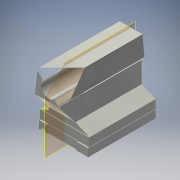
# Autodesk Inventor part: tail stock
Saved by Autodesk Inventor 2016 (Build 200138000, 138)
## iProperties
Created: 2017-02-14
Part Number: tail stock
Material: Steel
Document SubType Name: Modeling
Designer: m207653
Density: 7.85 g/cm^3
Appearance: Smooth - Ivory
Author: m207653
Autodesk Inventor part; units mm, degrees
ref_plane "YZ Plane" through (0, 0, 0) normal (1, 0, 0) x (0, 1, 0)
ref_plane "XZ Plane" through (0, 0, 0) normal (0, 1, 0) x (-1, 0, 0)
ref_plane "XY Plane" through (0, 0, 0) normal (0, 0, 1) x (1, 0, 0)
sketch "Sketch1" plane through (0, 0, 0) normal (0, 1, 0) x (-1, 0, 0)
  line L0 (-14.8781, 49.9341) -> (-14.8781, 23.9341)
  line L1 (-14.8781, 23.9341) -> (-165.8781, 23.9341)
  line L2 (-165.8781, 23.9341) -> (-165.8781, 49.9341)
  line L3 (-165.8781, 49.9341) -> (-14.8781, 49.9341)
  point P0 (0, 0)
  dimension "d19" = 26
  dimension "d20" = 151
  constraints: 8 end point, 3 perpendicular, 1 vertical
  measures "d19" distance of L0.start L0.end
  measures "d20" distance of L0.end L1.end
extrude "Extrusion1" add sketch "Sketch1" along normal blind 203
sketch "Sketch2" plane through (0, 0, 0) normal (0, -1, 0) x (1, 0, 0)
  line L0 (14.8781, 23.9341) -> (14.8781, 49.9341) projected
  line L1 (14.8781, 49.9341) -> (14.8781, 23.9341)
  line L2 (14.8781, 49.9341) -> (42.8781, 49.9341)
  line L3 (14.8781, 49.9341) -> (165.8781, 49.9341) projected
  line L4 (42.8781, 49.9341) -> (42.8781, 23.9341)
  line L5 (165.8781, 23.9341) -> (14.8781, 23.9341) projected
  line L6 (14.8781, 23.9341) -> (42.8781, 23.9341)
  line L7 (27.3781, 49.9341) -> (27.3781, 33.9341) construction
  line L8 (25.4781, 33.9341) -> (38.7147, 33.9341) construction
  line L9 (29.4781, 36.9341) -> (43.9589, 36.9341) construction
  line L10 (27.3781, 33.9341) -> (30.8781, 33.9341)
  line L11 (30.8781, 33.9341) -> (26.8781, 33.9341)
  line L12 (26.8781, 33.9341) -> (16.8781, 23.9341)
  line L13 (26.8781, 33.9341) -> (51.2693, 33.9341) construction
  line L14 (30.8781, 33.9341) -> (40.8781, 23.9341)
  line L15 (30.8781, 33.9341) -> (59.3837, 33.9341) construction
  point P0 (0, 0)
  dimension "d23" = 28
  dimension "d29" = 4
  dimension "d30" = 135
  dimension "d31" = 45
  dimension "d32" = 10
  dimension "d117" = 2
  constraints: 26 end point, 9 point on line, 4 horizontal, 2 collinear, 1 perpendicular
  measures "d23" distance of L0.end L2.end
  measures "d29" distance of L10.end L11.end
  measures "d30" angle of L12 L13
  measures "d31" angle of L14 L15
  measures "d32" vertical distance of L0.start L11.end
  measures "d117" distance of L0.start L12.end
extrude "Extrusion2" cut sketch "Sketch2" against normal through all contours L12 L11 L10 L14 L5
sketch "Sketch3" plane through (0, 0, 0) normal (0, -1, 0) x (1, 0, 0)
  line L0 (14.8781, 23.9341) -> (16.8781, 23.9341) projected
  line L1 (14.8781, 49.9341) -> (14.8781, 23.9341) projected
  line L2 (14.8781, 23.9341) -> (14.8781, 49.9341)
  line L3 (14.8781, 49.9341) -> (42.8781, 49.9341)
  line L4 (165.8781, 49.9341) -> (14.8781, 49.9341) projected
  line L5 (42.8781, 49.9341) -> (42.8781, 23.9341)
  line L6 (40.8781, 23.9341) -> (165.8781, 23.9341) projected
  line L7 (14.8781, 23.9341) -> (16.8781, 23.9341)
  line L8 (16.8781, 23.9341) -> (26.8781, 33.9341) projected
  line L9 (26.8781, 33.9341) -> (16.8781, 23.9341)
  line L10 (16.8781, 23.9341) -> (26.8781, 33.9341)
  line L11 (26.8781, 33.9341) -> (30.8781, 33.9341) projected
  line L12 (30.8781, 33.9341) -> (40.8781, 23.9341) projected
  line L13 (30.8781, 33.9341) -> (40.8781, 23.9341)
  line L14 (40.8781, 23.9341) -> (42.8781, 23.9341)
  point P0 (0, 0)
  dimension "d35" = 28
  constraints: 16 end point, 3 collinear, 2 point on line, 1 horizontal, 1 perpendicular, 1 vertical
  measures "d35" distance of L1.start L3.end
extrude "Extrusion3" add sketch "Sketch3" along normal blind 6
sketch "Sketch4" plane through (14.8781, 203, 49.9341) normal (0, 0, 1) x (1, 0, 0)
  line L0 (0, -209) -> (0, -203)
  line L1 (2, 0) -> (2, -209) projected
  line L2 (151, -203) -> (28, -203) projected
  line L3 (0, -203) -> (28, -203)
  line L4 (28, -209) -> (0, -209) projected
  line L5 (28, -203) -> (28, -209)
  line L6 (28, -209) -> (0, -209)
  line L7 (0, -209) -> (0, -203)
  point P0 (-14.8781, -203)
  constraints: 10 end point, 3 perpendicular, 1 collinear, 1 parallel
extrude "Extrusion4" cut sketch "Sketch4" against normal blind 2
sketch "Sketch5" plane through (0, 0, 0) normal (0, -1, 0) x (1, 0, 0)
  line L0 (165.8781, 23.9341) -> (40.8781, 23.9341) projected
  line L1 (165.8781, 23.9341) -> (165.8781, 47.9341)
  line L2 (165.8781, 49.9341) -> (165.8781, 23.9341) projected
  line L3 (42.8781, 47.9341) -> (14.8781, 47.9341) projected
  line L4 (165.8781, 47.9341) -> (128.8781, 47.9341)
  line L5 (128.8781, 47.9341) -> (128.8781, 23.9341)
  line L6 (165.8781, 23.9341) -> (128.8781, 23.9341)
  point P0 (0, 0)
  dimension "d40" = 37
  constraints: 8 end point, 3 perpendicular, 2 point on line, 1 collinear
  measures "d40" distance of L1.end L4.end
extrude "Extrusion5" add sketch "Sketch5" along normal blind 6
sketch "Sketch6" plane through (165.8781, 0, 49.9341) normal (1, 0, 0) x (0, 0, -1)
  line L0 (26, -6) -> (2, -6) projected
  line L1 (2, 0) -> (2, -6) projected
  line L2 (2, -6) -> (2, 0)
  line L3 (2, 0) -> (26, 0) projected
  line L4 (2, 0) -> (26, 0)
  line L5 (26, 0) -> (26, -6) projected
  line L6 (26, 0) -> (26, -6)
  line L7 (26, -6) -> (2, -6)
  line L8 (2, -6) -> (2, 0)
  point P0 (49.9341, 0)
  constraints: 10 end point, 4 collinear, 1 perpendicular
extrude "Extrusion6" add sketch "Sketch6" along normal blind 1
fillet "Fillet1" radius 5 2 edges at (166.8781, -3, 47.9341) (128.8781, -3, 47.9341)
sketch "Sketch8" plane through (14.8781, 0, 49.9341) normal (-1, 0, 0) x (0, 0, 1)
  line L0 (-2, -6) -> (-2, 0) projected
  line L1 (-26, 203) -> (-26, -6) projected
  line L2 (-2, -6) -> (-26, -6)
  line L3 (-26, -6) -> (-26, 0)
  line L4 (-2, 0) -> (0, 0) projected
  line L5 (-26, 0) -> (-2, 0)
  line L6 (-2, 0) -> (-2, -6)
  point P0 (-49.9341, 0)
  constraints: 8 end point, 4 perpendicular
extrude "Extrusion7" add sketch "Sketch8" along normal blind 1
fillet "Fillet3" radius 5 2 edges at (42.8781, -3, 47.9341) (13.8781, -3, 47.9341)
sketch "Sketch9" plane through (14.8781, 0, 49.9341) normal (0, 0, 1) x (1, 0, 0)
  line L0 (1, 202) -> (150, 202)
  line L1 (150, 202) -> (150, 1)
  line L2 (150, 1) -> (1, 1)
  line L3 (1, 1) -> (1, 202)
  line L4 (151, 203) -> (26, 203) projected
  line L5 (151, 0) -> (151, 203) projected
  line L6 (28, 0) -> (114, 0) projected
  line L7 (0, 203) -> (0, 0) projected
  point P0 (-14.8781, 0)
  dimension "d50" = 1
  dimension "d51" = 1
  dimension "d52" = 1
  dimension "d53" = 1
  constraints: 8 end point, 2 parallel, 1 horizontal, 1 perpendicular
  measures "d50" distance between parallel lines of L4 L0
  measures "d51" distance between parallel lines of L5 L1
  measures "d52" distance between parallel lines of L6 L2
  measures "d53" distance between parallel lines of L7 L3
extrude "Extrusion8" add sketch "Sketch9" along normal blind 1
sketch "Sketch10" plane through (14.8781, 0, 50.9341) normal (0, 0, 1) x (1, 0, 0)
  line L0 (0, 0) -> (0, 203) projected
  line L1 (0, 203) -> (151, 203) projected
  line L2 (0, 203) -> (151, 203)
  line L3 (151, 0) -> (151, 203) projected
  line L4 (151, 203) -> (151, 0)
  line L5 (151, 0) -> (0, 0)
  point P0 (-14.8781, 0)
  constraints: 6 end point, 2 perpendicular, 1 horizontal
extrude "Extrusion9" add sketch "Sketch10" along normal blind 26
sketch "Sketch11" plane through (14.8781, 0, 76.9341) normal (0, 0, 1) x (1, 0, 0)
  line L0 (151, 203) -> (0, 203) projected
  line L1 (0, 203) -> (151, 203)
  line L2 (151, 203) -> (151, -49)
  line L3 (151, -49) -> (0, -49)
  line L4 (0, -49) -> (0, 203)
  line L5 (0, 0) -> (151, 0) projected
  point P0 (-14.8781, 0)
  dimension "d58" = 49
  constraints: 8 end point, 2 parallel, 1 horizontal, 1 perpendicular
  measures "d58" distance between parallel lines of L3 L5
extrude "Extrusion10" add sketch "Sketch11" along normal blind 152
sketch "Sketch12" plane through (14.8781, -49, 76.9341) normal (0, -1, 0) x (1, 0, 0)
  line L0 (0, 0) -> (151, 0) projected
  line L1 (151, 152) -> (0, 152) projected
  line L2 (75.5, 152) -> (75.5, 0)
  line L3 (0, 0) -> (25.3832, 8.1737)
  line L4 (75.5, 152) -> (40.5, 152)
  line L5 (25.3832, 8.1737) -> (40.5, 152)
  line L6 (75.5, 152) -> (110.5, 152)
  line L7 (110.5, 152) -> (116.596, 94)
  line L8 (151, 0) -> (0, 0)
  line L9 (151, 0) -> (107.9707, 18.3787)
  line L10 (107.9707, 18.3787) -> (107.9707, 83.4635)
  line L11 (107.9707, 83.4635) -> (116.596, 94)
  line L12 (0, -26) -> (0, 152) projected
  line L13 (0, -26) -> (0, 0) projected
  line L14 (0, 152) -> (0, 0)
  line L15 (0, 152) -> (151, 152)
  line L16 (151, 0) -> (151, 152)
  point P0 (-14.8781, -76.9341)
  dimension "d61" = 35
  dimension "d62" = 35
  dimension "d63" = 96
  dimension "d64" = 96
  dimension "d65" = 58
  constraints: 26 end point, 2 midpoint, 2 point on line, 2 vertical, 1 collinear, 1 horizontal, 1 perpendicular
  measures "d61" distance of L2.start L4.end
  measures "d62" distance of L2.start L6.end
  measures "d63" angle of L1 L5
  measures "d64" angle of L1 L7
  measures "d65" vertical distance of L6.end L7.end
extrude "Extrusion11" cut sketch "Sketch12" against normal blind 295.5 contours L12 L1 L5 L3 | L9 L10 L11 L7 L1 L16
ref_plane "Work Plane1" through (90.3781, 0, 50.9341) normal (1, 0, 0) x (0, 0, -1)
sketch "Sketch13" plane through (90.3781, 0, 50.9341) normal (1, 0, 0) x (0, 0, -1)
  line L0 (-109.4635, -49) -> (-109.4635, 203) projected
  line L1 (-26, 0) -> (-109.4635, -49)
  line L2 (0, 0) -> (-26, 0) projected
  line L3 (-26, 0) -> (-26, -49)
  line L4 (-26, -49) -> (-106.0869, -49)
  line L5 (-178, -49) -> (-34.1737, -49) projected
  line L6 (-26, 0) -> (-106.0869, -49)
  line L7 (-44.3787, -49) -> (-44.3787, 203) projected
  line L8 (-44.3787, -11.2447) -> (-44.3787, -49)
  point P0 (50.9341, 0)
  constraints: 10 end point, 2 point on line, 1 collinear, 1 midpoint, 1 vertical, 1 other
extrude "Extrusion12" cut sketch "Sketch13" along normal mid plane 295.5 contours L7 L4 L6
sketch "Sketch14" plane through (90.3781, 0, 50.9341) normal (1, 0, 0) x (0, 0, -1)
  line L0 (-26, -49) -> (-44.3787, -49) projected
  line L1 (-44.3787, -49) -> (-26, -49)
  line L2 (-26, -49) -> (-44.3787, -49)
  line L3 (-44.3787, -49) -> (-44.3787, 0)
  line L4 (-26, 0) -> (-26, -49) projected
  line L5 (-44.3787, 0) -> (-26, 0)
  point P0 (50.9341, 0)
  constraints: 8 end point, 1 collinear, 1 horizontal, 1 perpendicular, 1 vertical
extrude "Extrusion13" cut sketch "Sketch14" along normal mid plane 295.5
sketch "Sketch15" plane through (90.3781, 0, 50.9341) normal (1, 0, 0) x (0, 0, -1)
  line L0 (-44.3787, 0) -> (-26, 0) projected
  line L1 (-106.0869, -49) -> (-44.3787, 0)
  line L2 (-106.0869, -49) -> (-44.3787, -11.2447) projected
  line L3 (-44.3787, 0) -> (-44.3787, -11.2447)
  line L4 (-44.3787, -11.2447) -> (-106.0869, -49)
  line L5 (-106.0869, -49) -> (-44.3787, -11.2447)
  line L6 (-44.3787, 0) -> (-44.3787, -11.2447)
  line L7 (-44.3787, 0) -> (-106.0869, -49)
  point P0 (50.9341, 0)
  constraints: 12 end point, 4 collinear, 1 perpendicular
extrude "Extrusion14" cut sketch "Sketch15" along normal mid plane 295.5
sketch "Sketch16" plane through (14.8781, 0, 50.9341) normal (0, -1, 0) x (1, 0, 0)
  line L0 (0, 0) -> (0, 26) projected
  line L1 (0, 26) -> (151, 26)
  line L2 (151, 26) -> (151, 0)
  line L3 (151, 0) -> (0, 0)
  line L4 (0, 0) -> (0, 26)
  point P0 (-14.8781, -50.9341)
  constraints: 8 end point, 2 perpendicular, 1 collinear, 1 horizontal
extrude "Extrusion15" add sketch "Sketch16" along normal blind 1
fillet "Fillet4" radius 2 1 edges at (90.3781, 0, 76.9341)
sketch "Sketch18" plane through (0, 0, 0) normal (0, -1, 0) x (1, 0, 0)
  line L0 (14.8781, 45.9341) -> (14.8781, 49.9341) projected
  line L1 (14.8781, 45.9341) -> (14.8781, 49.9341)
  line L2 (165.8781, 49.9341) -> (14.8781, 49.9341) projected
  line L3 (14.8781, 49.9341) -> (165.8781, 49.9341)
  line L4 (165.8781, 45.9341) -> (165.8781, 49.9341) projected
  line L5 (165.8781, 49.9341) -> (165.8781, 45.9341)
  line L6 (165.8781, 45.9341) -> (165.8781, 49.9341)
  arc A0 (165.8781, 45.9341) -> (161.8781, 47.9341) centre (161.8781, 42.9341) ccw projected
  arc A1 (161.8781, 47.9341) -> (165.8781, 45.9341) centre (161.8781, 42.9341) ccw
  arc A2 (133.8781, 47.9341) -> (128.8781, 42.9341) centre (133.8781, 42.9341) ccw projected
  line L7 (161.8781, 47.9341) -> (133.8781, 47.9341)
  arc A3 (133.8781, 47.9341) -> (128.8781, 42.9341) centre (133.8781, 42.9341) ccw
  line L8 (128.8781, 23.9341) -> (128.8781, 42.9341) projected
  line L9 (128.8781, 42.9341) -> (128.8781, 23.9341)
  line L10 (42.8781, 23.9341) -> (42.8781, 42.9341) projected
  line L11 (128.8781, 23.9341) -> (42.8781, 23.9341)
  line L12 (42.8781, 42.9341) -> (42.8781, 23.9341) projected
  line L13 (42.8781, 23.9341) -> (42.8781, 42.9341)
  arc A4 (42.8781, 42.9341) -> (37.8781, 47.9341) centre (37.8781, 42.9341) ccw projected
  arc A5 (42.8781, 42.9341) -> (37.8781, 47.9341) centre (37.8781, 42.9341) ccw
  line L14 (18.8781, 47.9341) -> (37.8781, 47.9341) projected
  line L15 (37.8781, 47.9341) -> (18.8781, 47.9341)
  line L16 (14.8781, 23.9341) -> (14.8781, 45.9341) projected
  arc A6 (18.8781, 47.9341) -> (14.8781, 45.9341) centre (18.8781, 42.9341) ccw
  point P0 (0, 0)
  constraints: 18 end point, 8 point on circle, 4 centre point, 4 collinear, 3 perpendicular, 2 concentric, 2 horizontal, 2 tangent
extrude "Extrusion16" add sketch "Sketch18" along normal blind 1 contours L0 L2 L4 A0 L7 A2 L8 L11 L10 A4 L14 A6
sketch "Sketch19" plane through (55.3781, -49, 228.9341) normal (0, -1, 0) x (1, 0, 0)
  circle A0 centre (35, -37.3579) radius 25
  point P0 (-55.3781, -228.9341)
  dimension "d87" = 50
  constraints: 1 centre point
  measures "d87" diameter of A0
extrude "Extrusion17" cut sketch "Sketch19" against normal blind 300
ref_plane "Work Plane2" through (30.8781, -6, 33.9341) normal (0, -1, 0) x (1, 0, 0)
sketch "Sketch20" plane through (30.8781, -6, 33.9341) normal (0, -1, 0) x (1, 0, 0)
  line L0 (-17, -10) -> (-17, 16)
  line L1 (135, 16) -> (-16, 16) projected
  line L2 (-17, 16) -> (136, 16)
  line L3 (135, -10) -> (136, -10) projected
  line L4 (136, 16) -> (136, -10)
  line L5 (136, -10) -> (-17, -10)
  line L6 (98, -10) -> (136, -10) projected
  point P0 (-30.8781, -33.9341)
  constraints: 8 end point, 3 perpendicular, 1 collinear
extrude "Extrusion18" cut sketch "Sketch20" against normal blind 5
sketch "Sketch21" plane through (166.8781, 0, 49.9341) normal (1, 0, 0) x (0, 0, -1)
  line L0 (7, -1) -> (26, -1) projected
  line L1 (26, -1) -> (26, 0) projected
  line L2 (26, -1) -> (26, 0)
  line L3 (4, 0) -> (7, 0) projected
  line L4 (26, 0) -> (4, 0)
  line L5 (4, 0) -> (4, -1) projected
  line L6 (4, 0) -> (4, -1)
  line L7 (4, -1) -> (26, -1)
  point P0 (49.9341, 0)
  constraints: 8 end point, 2 collinear, 1 perpendicular, 1 vertical
extrude "Extrusion19" cut sketch "Sketch21" against normal blind 1
sketch "Sketch23" plane through (13.8781, 0, 49.9341) normal (-1, 0, 0) x (0, 0, 1)
  line L0 (-26, 0) -> (-4, 0) projected
  line L1 (-26, 203) -> (-26, -1) projected
  line L2 (-26, 0) -> (-26, -1)
  line L3 (0, -1) -> (-4, -1) projected
  line L4 (-26, -1) -> (-4, -1)
  line L5 (-4, -1) -> (-4, 0) projected
  line L6 (-4, -1) -> (-4, 0)
  line L7 (-4, 0) -> (-26, 0)
  point P0 (-49.9341, 0)
  constraints: 8 end point, 2 collinear, 2 perpendicular
extrude "Extrusion20" cut sketch "Sketch23" against normal blind 1
sketch "Sketch24" plane through (0, -1, 0) normal (0, -1, 0) x (1, 0, 0)
  line L0 (14.8781, 49.9341) -> (14.8781, 23.9341) projected
  line L1 (14.8781, 25.9341) -> (165.8781, 25.9341)
  line L2 (165.8781, 23.9341) -> (165.8781, 49.9341) projected
  line L3 (165.8781, 23.9341) -> (40.8781, 23.9341) projected
  line L4 (14.8781, 25.9341) -> (14.8781, 23.9341)
  line L5 (14.8781, 25.9341) -> (14.8781, 23.9341)
  line L6 (14.8781, 23.9341) -> (165.8781, 23.9341)
  line L7 (165.8781, 23.9341) -> (165.8781, 25.9341)
  point P0 (0, 0)
  dimension "d96" = 2
  constraints: 10 end point, 3 collinear, 2 point on line, 1 horizontal, 1 perpendicular
  measures "d96" distance between parallel lines of L3 L1
extrude "Extrusion21" cut sketch "Sketch24" against normal blind 207
sketch "Sketch25" plane through (0, -1, 0) normal (0, -1, 0) x (1, 0, 0)
  line L0 (14.8781, 25.9341) -> (14.8781, 49.9341) projected
  line L1 (14.8781, 49.9341) -> (14.8781, 25.9341)
  line L2 (14.8781, 25.9341) -> (43.5711, 25.9341)
  line L3 (43.5711, 25.9341) -> (43.5711, 49.9341)
  line L4 (14.8781, 49.9341) -> (165.8781, 49.9341) projected
  line L5 (14.8781, 49.9341) -> (43.5711, 49.9341)
  point P0 (0, 0)
  constraints: 8 end point, 2 collinear, 2 perpendicular, 1 point on line
extrude "Extrusion22" add sketch "Sketch25" against normal blind 204
sketch "Sketch26" plane through (0, -1, 0) normal (0, -1, 0) x (1, 0, 0)
  line L0 (165.8781, 25.9341) -> (17.7541, 25.9341)
  line L1 (165.8781, 25.9341) -> (14.8781, 25.9341) projected
  line L2 (17.7541, 25.9341) -> (25.5677, 32.4905)
  line L3 (17.7541, 25.9341) -> (27.9541, 25.9341) construction
  line L4 (29.3677, 32.4905) -> (37.1814, 25.9341)
  line L5 (25.5677, 32.4905) -> (26.8048, 33.5286)
  line L6 (26.8048, 33.5286) -> (28.1307, 33.5286)
  line L7 (28.1307, 33.5286) -> (29.3677, 32.4905)
  point P0 (0, 0)
  dimension "d101" = 148.124
  dimension "d102" = 10.2
  dimension "d103" = 40
  dimension "d104" = 3.8
  constraints: 14 end point, 3 point on line, 2 horizontal, 1 equal length
  measures "d101" distance of L0.start L0.end
  measures "d102" distance of L0.end L2.end
  measures "d103" angle of L3 L2
  measures "d104" distance of L2.end L4.start
extrude "Extrusion23" cut sketch "Sketch26" against normal blind 204
sketch "Sketch27" plane through (0, -1, 0) normal (0, -1, 0) x (1, 0, 0)
  line L0 (14.8781, 25.9341) -> (14.8781, 49.9341) projected
  line L1 (14.8781, 25.9341) -> (14.8781, 49.9341)
  line L2 (14.8781, 49.9341) -> (165.8781, 49.9341) projected
  line L3 (40.1781, 49.9341) -> (40.1781, 25.9341)
  line L4 (40.1781, 25.9341) -> (37.1814, 25.9341)
  line L5 (37.1814, 25.9341) -> (28.1307, 33.5286) projected
  line L6 (37.1814, 25.9341) -> (28.1307, 33.5286)
  line L7 (26.8048, 33.5286) -> (17.7541, 25.9341) projected
  line L8 (28.1307, 33.5286) -> (26.8048, 33.5286)
  line L9 (17.7541, 25.9341) -> (14.8781, 25.9341) projected
  line L10 (26.8048, 33.5286) -> (17.7541, 25.9341)
  line L11 (17.7541, 25.9341) -> (14.8781, 25.9341)
  line L12 (14.8781, 49.5118) -> (40.1781, 49.5118)
  point P0 (0, 0)
  dimension "d108" = 25.3
  constraints: 16 end point, 4 collinear, 3 perpendicular, 3 point on line
  measures "d108" distance of L0.end L3.start
extrude "Extrusion24" add sketch "Sketch27" along normal blind 3 contours L0 L12 L3 L4 L5 L8 L7 L9
fillet "Fillet5" radius 3 1 edges at (14.8781, -2.5, 49.5118)
fillet "Fillet6" radius 3 1 edges at (40.1781, -2.5, 49.5118)
sketch "Sketch28" plane through (0, -1, 0) normal (0, -1, 0) x (1, 0, 0)
  line L0 (40.1781, 25.9341) -> (165.8781, 25.9341) projected
  line L1 (165.8781, 25.9341) -> (165.8781, 49.5118)
  line L2 (165.8781, 25.9341) -> (165.8781, 49.9341) projected
  line L3 (17.8781, 49.5118) -> (37.1781, 49.5118) projected
  line L4 (165.8781, 49.5118) -> (129.6781, 49.5118)
  line L5 (129.6781, 49.5118) -> (129.6781, 25.9341)
  point P0 (0, 0)
  dimension "d113" = 36.2
  constraints: 6 end point, 2 perpendicular, 2 point on line, 1 horizontal
  measures "d113" distance of L1.end L4.end
extrude "Extrusion25" add sketch "Sketch28" along normal blind 3
fillet "Fillet7" radius 3 2 edges at (165.8781, -2.5, 49.5118) (129.6781, -2.5, 49.5118)
body "Solid1"
